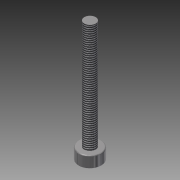
# Autodesk Inventor part: AdjBolt
Saved by Autodesk Inventor 2015 (Build 190159000, 159)
## iProperties
Created: 2018-03-01
Part Number: AdjBolt
Material: Stainless Steel
Document SubType Name: Modeling
Designer: Silas
Density: 8 g/cm^3
Appearance: Semi-Polished
Author: Silas
Autodesk Inventor part; units mm, degrees
ref_plane "YZ Plane" through (0, 0, 0) normal (1, 0, 0) x (0, 1, 0)
ref_plane "XZ Plane" through (0, 0, 0) normal (0, 1, 0) x (-1, 0, 0)
ref_plane "XY Plane" through (0, 0, 0) normal (0, 0, 1) x (1, 0, 0)
sketch "Sketch1" plane through (0, 0, 0) normal (0, 0, 1) x (1, 0, 0)
  circle A0 centre (0, 0) radius 1.5
  dimension "d0" = 3
  constraints: 1 centre point, 1 coincident
  measures "d0" diameter of A0
extrude "Extrusion1" add sketch "Sketch1" along normal blind 28.8
thread "Thread1" size "M3x0.5" class "6g" standard "ANSI Metric M Profile" full length
sketch "Sketch2" plane through (0, 0, 0) normal (0, 0, -1) x (-1, 0, 0)
  circle A0 centre (0, 0) radius 3
  dimension "d5" = 6
  constraints: 1 centre point, 1 coincident
  measures "d5" diameter of A0
extrude "Extrusion2" add sketch "Sketch2" along normal blind 3
sketch "Sketch3" plane through (0, 0, -3) normal (0, 0, -1) x (-1, 0, 0)
  circle A0 centre (0, 0) radius 1.5 projected
  line L0 (0, -2.3094) -> (-2, -1.1547)
  line L1 (-2, -1.1547) -> (-2, 1.1547)
  line L2 (-2, 1.1547) -> (0, 2.3094)
  line L3 (0, 2.3094) -> (2, 1.1547)
  line L4 (2, 1.1547) -> (2, -1.1547)
  line L5 (2, -1.1547) -> (0, -2.3094)
  dimension "d8" = 2
  constraints: 12 end point, 1 coincident, 13 other
  measures "d8" distance from line of L1 point (0, 0)
extrude "Extrusion3" cut sketch "Sketch3" against normal blind 1.5 contours A0 | L0 L1 L2 L3 L4 L5
fillet "Fillet1" radius 0.25 8 edges at (3, 0, 0) (3, 0, -3) (-1, -1.7321, -3) (-2, 0, -3) (-1, 1.7321, -3) (1, 1.7321, -3) (2, 0, -3) (1, -1.7321, -3)
body "Solid1"
